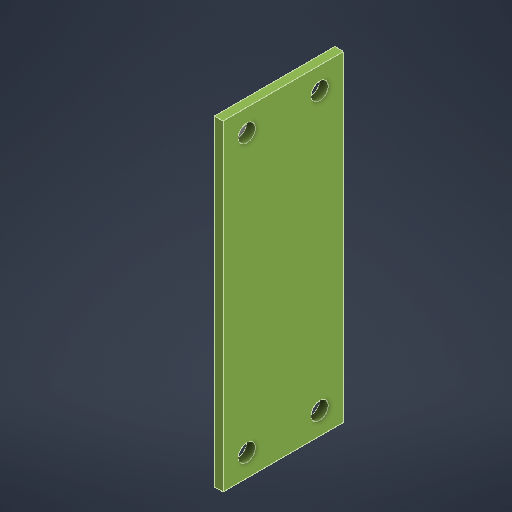
# Autodesk Inventor part: bus_connector_board
Saved by Autodesk Inventor 2025 (Build 290162000, 162)
## iProperties
Created: 2024-09-04
Part Number: bus_connector_board
Material: Generic
Document SubType Name: Modeling
Designer: Dawid
Density: 1 g/cm^3
Appearance: Default
Author: Dawid
Autodesk Inventor part; units mm, degrees
ref_plane "YZ Plane" through (0, 0, 0) normal (1, 0, 0) x (0, 1, 0)
ref_plane "XZ Plane" through (0, 0, 0) normal (0, 1, 0) x (-1, 0, 0)
ref_plane "XY Plane" through (0, 0, 0) normal (0, 0, 1) x (1, 0, 0)
sketch "Sketch1" plane through (0, 0, 0) normal (1, 0, 0) x (0, 1, 0)
  line L0 (0, 0) -> (56, 0)
  line L1 (56, 0) -> (56, -21)
  line L2 (56, -21) -> (0, -21)
  line L3 (0, -21) -> (0, 0)
  circle A0 centre (52.13, -4.15) radius 1.5
  circle A1 centre (52.13, -16.85) radius 1.5
  circle A2 centre (3.87, -4.15) radius 1.5
  circle A3 centre (3.87, -16.85) radius 1.5
  line L4 (52.13, -4.15) -> (3.87, -16.85) construction
  point P0 (28, -10.5)
  point P1 (0, -10.5)
  point P2 (28, 0)
  dimension "d0" = 21
  dimension "d1" = 56
  dimension "d2" = 12.7
  dimension "d3" = 48.26
  dimension "d4" = 3
  constraints: 10 end point, 4 centre point, 3 equal radius, 3 horizontal alignment, 3 midpoint, 3 vertical alignment, 2 parallel, 1 horizontal, 1 perpendicular
  measures "d0" distance of L0.end L1.end
  measures "d1" distance of L1.end L2.end
  measures "d2" distance of L4.start A1.centre
  measures "d3" distance of L4.end A1.centre
  measures "d4" diameter of A0
extrude "Extrusion1" add sketch "Sketch1" along normal blind 1.5
sketch "Sketch2" plane through (0, 0, 0) normal (-1, 0, 0) x (0, 0, 1)
  line L0 (-21, 0) -> (-21, 56) construction
  line L1 (0, 0) -> (-21, 0) construction
  line L2 (0, 56) -> (0, 0) construction
  line L3 (-21, 56) -> (0, 56) construction
  circle A0 centre (-16.85, 3.87) radius 1.5 construction
  circle A1 centre (-4.15, 3.87) radius 1.5 construction
  circle A2 centre (-16.85, 52.13) radius 1.5 construction
  circle A3 centre (-4.15, 52.13) radius 1.5 construction
  line L4 (-13.04, 46) -> (-7.96, 46)
  line L5 (-7.96, 46) -> (-7.96, 10)
  line L6 (-7.96, 10) -> (-13.04, 10)
  line L7 (-13.04, 10) -> (-13.04, 46)
  line L8 (-16.85, 52.13) -> (-4.15, 3.87) construction
  point P0 (-10.5, 28)
  point P1 (-13.04, 28)
  point P2 (-10.5, 10)
  dimension "d7" = 5.08
  dimension "d8" = 36
  constraints: 10 end point, 3 midpoint, 2 parallel, 1 horizontal, 1 horizontal alignment, 1 perpendicular, 1 vertical alignment
  measures "d7" distance of L4.start L4.end
  measures "d8" distance of L4.end L5.end
extrude "Extrusion2" add sketch "Sketch2" along normal blind 8 separate body
sketch "Sketch3" plane through (-8, 0, 0) normal (-1, 0, 0) x (0, 0, 1)
  line L0 (-13.04, 10) -> (-7.96, 10) projected
  line L1 (-7.96, 10) -> (-7.96, 46) projected
  line L2 (-7.96, 46) -> (-13.04, 46) projected
  line L3 (-13.04, 46) -> (-13.04, 10) projected
  line L4 (-12.27, 45.23) -> (-11.27, 45.23)
  line L5 (-11.27, 45.23) -> (-11.27, 44.23)
  line L6 (-11.27, 44.23) -> (-12.27, 44.23)
  line L7 (-12.27, 44.23) -> (-12.27, 45.23)
  line L8 (-12.27, 45.23) -> (-11.27, 44.23) construction
  point P0 (0, 0)
  point P1 (-11.77, 44.73)
  dimension "d11" = 1.27
  dimension "d12" = 1.27
  dimension "d13" = 1
  constraints: 10 end point, 2 parallel, 2 perpendicular, 1 horizontal, 1 midpoint
  measures "d11" distance from line of L2 point (-11.77, 44.73)
  measures "d12" distance from line of L3 point (-11.77, 44.73)
  measures "d13" distance of L5.end L6.end
extrude "Extrusion3" cut sketch "Sketch3" against normal blind 3 contours L4 L5 L6 L7 bodies 2
chamfer "Chamfer1" distance 0.2 angle 45 4 edges at (-5, 44.73, -12.27) (-5, 44.23, -11.77) (-5, 45.23, -11.77) (-5, 44.73, -11.27)
pattern_linear "Rectangular Pattern1" count 14 spacing 2.54 along (0, -1, 0) count 2 spacing 2.54 along (0, 0, 1) of "Extrusion3", "Chamfer1" bodies 2
